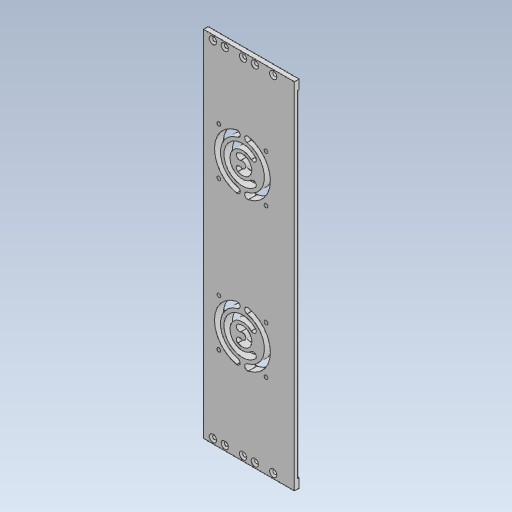
# Autodesk Inventor part: rIGHTbOXcOVER
Saved by Autodesk Inventor 2020 (Build 240168000, 168)
## iProperties
Created: 2019-06-04
Part Number: rIGHTbOXcOVER
Material: Generic
Document SubType Name: Modeling
Designer: LillaHunden
Density: 1 g/cm^3
Appearance: Default
Author: LillaHunden
Autodesk Inventor part; units mm, degrees
ref_plane "YZ Plane" through (0, 0, 0) normal (1, 0, 0) x (0, 1, 0)
ref_plane "XZ Plane" through (0, 0, 0) normal (0, 1, 0) x (-1, 0, 0)
sketch "Sketch1" plane through (0, 0, 0) normal (0, 0, 1) x (1, 0, 0)
  line L0 (0, -288) -> (0, 12) projected
  line L1 (0, 12) -> (76.9823, 12) projected
  line L2 (76.9823, 12) -> (76.9823, -288) projected
  line L3 (76.9823, -288) -> (0, -288) projected
  circle A0 centre (18, -283.95) radius 3.15 projected
  circle A1 centre (43.4912, -283.95) radius 3.15 projected
  circle A2 centre (68.9823, -283.95) radius 3.15 projected
  circle A3 centre (58.9823, -283.95) radius 3.15 projected
  circle A4 centre (33.4912, -283.95) radius 3.15 projected
  circle A5 centre (8, -283.95) radius 3.15 projected
  circle A6 centre (18, 7.95) radius 3.15 projected
  circle A7 centre (43.4912, 7.95) radius 3.15 projected
  circle A8 centre (68.9823, 7.95) radius 3.15 projected
  circle A9 centre (33.4912, 7.95) radius 3.15 projected
  circle A10 centre (8, 7.95) radius 3.15 projected
  circle A11 centre (58.9823, 7.95) radius 3.15 projected
  circle A12 centre (51.5, -236.7541) radius 3.15 projected
  circle A13 centre (51.5, -186.7541) radius 3.15 projected
  circle A14 centre (61.5, -161.7541) radius 3.15 projected
  circle A15 centre (61.5, -186.7541) radius 3.15 projected
  circle A16 centre (61.5, -211.7541) radius 3.15 projected
  circle A17 centre (51.5, -161.7541) radius 3.15 projected
  circle A18 centre (51.5, -211.7541) radius 3.15 projected
  circle A19 centre (51.5, -261.7541) radius 3.15 projected
  point P0 (0, 0)
extrude "Extrusion1" add sketch "Sketch1" along normal blind 12 contours L0 L1 L2 L3 | A0 | A1 | A2 | A3 | A4 | A5 | A6 | A7 | A8 | A9 | A10 | A11 | A12 | A13 | A14 | A15 | A16 | A17 | A18 | A19
sketch "Sketch2" plane through (0, 0, 0) normal (0, 0, -1) x (-1, 0, 0)
  line L0 (-67, 4) -> (-76.9823, 4) construction
  line L1 (-76.9823, -280) -> (-76.9823, 4) construction
  line L2 (-67, -280) -> (-76.9823, -280) construction
  line L3 (-67, 4) -> (-67, -280) construction
  line L4 (-66.8, -280.2) -> (-77.1823, -280.2)
  line L5 (-77.1823, -280.2) -> (-77.1823, 4.2)
  line L6 (-77.1823, 4.2) -> (-66.8, 4.2)
  line L7 (-66.8, 4.2) -> (-66.8, -280.2)
  point P0 (0, 0)
  dimension "d2" = 0.2
  constraints: 8 end point, 3 other
  measures "d2" distance between parallel lines of L3 L7
extrude "Extrusion2" cut sketch "Sketch2" against normal blind 9.25
sketch "Sketch3" plane through (0, 0, 0) normal (0, 0, -1) x (-1, 0, 0)
  line L0 (0, -276) -> (-67, -276) construction
  line L1 (-76.9823, -288) -> (0, -288) construction
  line L2 (-76.9823, -280) -> (-76.9823, -288) construction
  line L3 (-67, -280) -> (-67, 4) construction
  line L4 (-76.9823, -288) -> (0, -288)
  line L5 (0, -288) -> (0, -275.8)
  line L6 (0, -275.8) -> (-76.9823, -275.8)
  line L7 (-76.9823, -275.8) -> (-76.9823, -288)
  line L8 (0, 12) -> (0, -288) projected
  point P0 (0, 0)
  point P1 (0, -281.9)
  dimension "d5" = 0.2
  constraints: 8 end point, 2 parallel, 1 horizontal, 1 midpoint, 1 perpendicular, 1 point on line
  measures "d5" distance between parallel lines of L0 L6
extrude "Extrusion3" cut sketch "Sketch3" against normal blind 8.05
sketch "Sketch4" plane through (66.8, -280.2, 9.25) normal (1, 0, 0) x (0, 0, -1)
  line L0 (1.2, 4.4) -> (9.25, 4.4) construction
  line L1 (9.25, 284.4) -> (9.25, 4.4) construction
  line L2 (9.25, 284.4) -> (0, 284.4) projected
  line L3 (0, 284.4) -> (0, 0) projected
  line L4 (1.2, 0) -> (0, 0) projected
  line L5 (1.2, 0) -> (1.2, 4.4) projected
  line L6 (1.25, 284.2) -> (1.25, 0.2) projected
  line L7 (1.25, 284.2) -> (1.25, 284.4)
  line L8 (0, 284.4) -> (1.2, 284.4)
  line L9 (1.2, 284.4) -> (1.2, 0)
  line L10 (1.2, 0) -> (0, 0)
  line L11 (0, 0) -> (0, 284.4)
  point P0 (9.25, 280.2)
  constraints: 10 end point, 2 parallel, 2 perpendicular, 1 horizontal, 1 point on line
extrude "Extrusion4" add sketch "Sketch4" along normal blind 9
sketch "Sketch5" plane through (0, 0, 0) normal (0, 0, -1) x (-1, 0, 0)
  line L0 (0, 0) -> (-67, 0) construction
  line L1 (-75.8, 4.2) -> (-66.8, 4.2) construction
  line L2 (-66.8, 4.2) -> (-66.8, -275.8) construction
  line L3 (-76.9823, 4.2) -> (-66.8, 4.2) construction
  line L4 (-76.9823, 4.2) -> (-76.9823, 12) construction
  line L5 (-76.9823, 12) -> (0, 12) construction
  line L6 (0, 12) -> (0, -275.8) construction
  line L7 (0, -0.2) -> (-67, -0.2)
  line L8 (-76.9823, 12) -> (0, 12)
  line L9 (0, 12) -> (0, -0.2)
  line L10 (0, -0.2) -> (-76.9823, -0.2)
  line L11 (-76.9823, -0.2) -> (-76.9823, 12)
  dimension "d10" = 0.2
  constraints: 10 end point, 3 parallel, 1 horizontal, 1 perpendicular
  measures "d10" distance between parallel lines of L0 L7
ref_plane "Work Plane1" through (0, 0, 8) normal (0, 0, 1) x (1, 0, 0)
extrude "Extrusion5" cut sketch "Sketch5" against normal up to surface (8 mm away)
sketch "Sketch6" plane through (0, -0.2, 0) normal (0, 1, 0) x (1, 0, 0)
  point P0 (56.9823, -3)
  point P1 (46.9823, -3)
  point P2 (30, -3)
  point P3 (20, -3)
hole "Hole1" at (56.9823, -0.2, 3) at (46.9823, -0.2, 3) at (30, -0.2, 3) at (20, -0.2, 3) direction (0, -1, 0) diameter 2.459 depth 8 tip angle 120 thread size "M3x0.5" class "6H" standard "ISO Metric profile"
sketch "Sketch7" plane through (0, 0, 12) normal (0, 0, 1) x (1, 0, 0)
  circle A0 centre (68.9823, 7.95) radius 3.15 construction
  circle A1 centre (58.9823, 7.95) radius 3.15 construction
  circle A2 centre (43.4912, 7.95) radius 3.15 construction
  circle A3 centre (33.4912, 7.95) radius 3.15 construction
  circle A4 centre (18, 7.95) radius 3.15 construction
  circle A5 centre (8, 7.95) radius 3.15 construction
  circle A6 centre (8, -283.95) radius 3.15 construction
  circle A7 centre (18, -283.95) radius 3.15 construction
  circle A8 centre (33.4912, -283.95) radius 3.15 construction
  circle A9 centre (43.4912, -283.95) radius 3.15 construction
  circle A10 centre (58.9823, -283.95) radius 3.15 construction
  circle A11 centre (68.9823, -283.95) radius 3.15 construction
  point P0 (0, 0)
sketch "Sketch9" plane through (0, 0, 12) normal (0, 0, 1) x (1, 0, 0)
  point P0 (8, 7.95)
  point P1 (18, 7.95)
  point P2 (33.4912, 7.95)
  point P3 (43.4912, 7.95)
  point P4 (58.9823, 7.95)
hole "Hole4" at (8, 7.95, 12) at (18, 7.95, 12) at (33.4912, 7.95, 12) at (43.4912, 7.95, 12) at (58.9823, 7.95, 12) direction (0, 0, -1) diameter 3.4 depth 4 countersink diameter 6.3 countersink angle 90
sketch "Sketch10" plane through (0, 0, 12) normal (0, 0, 1) x (1, 0, 0)
  point P0 (58.9823, -283.95)
  point P1 (43.4912, -283.95)
  point P2 (33.4912, -283.95)
  point P3 (18, -283.95)
  point P4 (8, -283.95)
hole "Hole6" at (58.9823, -283.95, 12) at (43.4912, -283.95, 12) at (33.4912, -283.95, 12) at (18, -283.95, 12) at (8, -283.95, 12) direction (0, 0, -1) diameter 3.4 depth 3.95 countersink diameter 6.3 countersink angle 90
sketch "Sketch11" plane through (0, 0, 12) normal (0, 0, 1) x (1, 0, 0)
  line L0 (53, -176.5677) -> (13, -176.5677) construction
  line L1 (13, -176.5677) -> (13, -216.5677) construction
  line L2 (13, -216.5677) -> (53, -216.5677) construction
  line L3 (53, -216.5677) -> (53, -176.5677) construction
  line L4 (53, -50.8348) -> (13, -50.8348) construction
  line L5 (13, -50.8348) -> (13, -90.8348) construction
  line L6 (13, -90.8348) -> (53, -90.8348) construction
  line L7 (53, -90.8348) -> (53, -50.8348) construction
  line L8 (0, 12) -> (0, -288) projected
  point P0 (0, 0)
  point P1 (53, -70.8348)
  point P2 (53, -196.5677)
  dimension "d41" = 40
  dimension "d42" = 40
  dimension "d43" = 40
  dimension "d44" = 40
  dimension "d45" = 13
  constraints: 16 end point, 8 coincident, 4 parallel, 2 horizontal, 2 midpoint, 2 perpendicular, 1 vertical alignment
  measures "d41" distance of L2.end L1.end
  measures "d42" distance of L1.end L0.end
  measures "d43" distance of L6.end L5.end
  measures "d44" distance of L5.end L4.end
  measures "d45" distance between parallel lines of L8 L5
hole "Hole8" at (13, -176.5677, 12) at (13, -216.5677, 12) at (53, -216.5677, 12) at (53, -176.5677, 12) at (13, -50.8348, 12) at (13, -90.8348, 12) at (53, -90.8348, 12) at (53, -50.8348, 12) direction (0, 0, -1) diameter 3.242 end through all thread size "M4x0.7" class "6H" standard "ISO Metric profile"
sketch "Sketch12" plane through (0, 0, 12) normal (0, 0, 1) x (1, 0, 0)
  circle A0 centre (53, -90.8348) radius 1.621 construction
  circle A1 centre (13, -50.8348) radius 1.621 construction
  circle A2 centre (53, -216.5677) radius 1.621 construction
  circle A3 centre (13, -176.5677) radius 1.621 construction
  circle A4 centre (13, -216.5677) radius 1.621 construction
  circle A5 centre (53, -176.5677) radius 1.621 construction
  circle A6 centre (13, -90.8348) radius 1.621 construction
  circle A7 centre (53, -50.8348) radius 1.621 construction
  circle A8 centre (18, -283.95) radius 3.15 construction
  circle A9 centre (43.4912, -283.95) radius 3.15 construction
  circle A10 centre (58.9823, -283.95) radius 3.15 construction
  circle A11 centre (33.4912, -283.95) radius 3.15 construction
  circle A12 centre (8, -283.95) radius 3.15 construction
  circle A13 centre (43.4912, 7.95) radius 3.15 construction
  circle A14 centre (18, 7.95) radius 3.15 construction
  circle A15 centre (8, 7.95) radius 3.15 construction
  circle A16 centre (33.4912, 7.95) radius 3.15 construction
  circle A17 centre (58.9823, 7.95) radius 3.15 construction
  line L0 (76.9823, 12) -> (0, 12) construction
  line L1 (0, 12) -> (0, -288) construction
  line L2 (0, -288) -> (76.9823, -288) construction
  line L3 (76.9823, -288) -> (76.9823, 12) construction
  line L4 (53, -90.8348) -> (13, -50.8348) construction
  line L5 (13, -50.8348) -> (53, -50.8348) construction
  line L6 (53, -50.8348) -> (13, -90.8348) construction
  line L7 (13, -176.5677) -> (13, -216.5677) construction
  line L8 (13, -216.5677) -> (53, -216.5677) construction
  line L9 (53, -216.5677) -> (13, -176.5677) construction
  line L10 (53, -176.5677) -> (13, -216.5677) construction
  circle A18 centre (33, -70.8348) radius 24 construction
  circle A19 centre (33, -196.5677) radius 24 construction
  arc A20 (37.3584, -91.5413) -> (37.3584, -50.1283) centre (33, -70.8348) ccw construction
  arc A21 (37.8806, -94.0225) -> (37.8806, -47.647) centre (33, -70.8348) ccw
  arc A22 (36.8361, -89.06) -> (36.8361, -52.6095) centre (33, -70.8348) ccw
  arc A23 (36.8361, -89.06) -> (37.8806, -94.0225) centre (37.3584, -91.5413) ccw
  arc A24 (37.8806, -47.647) -> (36.8361, -52.6095) centre (37.3584, -50.1283) ccw
  arc A25 (42.3123, -61.5224) -> (42.3123, -80.1471) centre (33, -70.8348) ccw construction
  arc A26 (44.1052, -59.7295) -> (44.1052, -81.94) centre (33, -70.8348) ccw
  arc A27 (40.5194, -63.3154) -> (40.5194, -78.3541) centre (33, -70.8348) ccw
  arc A28 (40.5194, -63.3154) -> (44.1052, -59.7295) centre (42.3123, -61.5224) ccw
  arc A29 (44.1052, -81.94) -> (40.5194, -78.3541) centre (42.3123, -80.1471) ccw
  line L11 (33, -43.5046) -> (33, -109.6187) construction
  line L12 (53, -50.8348) -> (13, -50.8348) construction
  circle A30 centre (33, -70.8348) radius 24 construction
  arc A31 (28.6416, -50.1283) -> (28.6416, -91.5413) centre (33, -70.8348) ccw construction
  arc A32 (28.1194, -47.647) -> (28.1194, -94.0225) centre (33, -70.8348) ccw
  arc A33 (29.1639, -52.6095) -> (29.1639, -89.06) centre (33, -70.8348) ccw
  arc A34 (28.1194, -94.0225) -> (29.1639, -89.06) centre (28.6416, -91.5413) ccw
  arc A35 (29.1639, -52.6095) -> (28.1194, -47.647) centre (28.6416, -50.1283) ccw
  arc A36 (30.3412, -75.5506) -> (30.3412, -66.1189) centre (33, -70.8348) ccw construction
  arc A37 (29.0751, -77.7962) -> (29.0751, -63.8734) centre (33, -70.8348) ccw
  arc A38 (31.6072, -73.3051) -> (31.6072, -68.3644) centre (33, -70.8348) ccw
  arc A39 (31.6072, -73.3051) -> (29.0751, -77.7962) centre (30.3412, -75.5506) ccw
  arc A40 (29.0751, -63.8734) -> (31.6072, -68.3644) centre (30.3412, -66.1189) ccw
  arc A41 (28.1194, -219.7555) -> (29.1639, -214.793) centre (28.6416, -217.2743) ccw
  arc A42 (44.1052, -207.673) -> (40.5194, -204.0871) centre (42.3123, -205.8801) ccw
  arc A43 (29.0751, -203.5292) -> (29.0751, -189.6064) centre (33, -196.5678) ccw
  arc A44 (29.0751, -189.6064) -> (31.6072, -194.0974) centre (30.3412, -191.8519) ccw
  arc A45 (40.5194, -189.0484) -> (40.5194, -204.0871) centre (33, -196.5678) ccw
  arc A46 (37.8806, -173.38) -> (36.8361, -178.3425) centre (37.3584, -175.8613) ccw
  arc A47 (42.3123, -187.2554) -> (42.3123, -205.8801) centre (33, -196.5678) ccw construction
  arc A48 (29.1639, -178.3425) -> (28.1194, -173.38) centre (28.6416, -175.8613) ccw
  arc A49 (36.8361, -214.793) -> (36.8361, -178.3425) centre (33, -196.5678) ccw
  arc A50 (44.1052, -185.4625) -> (44.1052, -207.673) centre (33, -196.5678) ccw
  arc A51 (37.3584, -217.2743) -> (37.3584, -175.8613) centre (33, -196.5678) ccw construction
  arc A52 (29.1639, -178.3425) -> (29.1639, -214.793) centre (33, -196.5678) ccw
  arc A53 (37.8806, -219.7555) -> (37.8806, -173.38) centre (33, -196.5678) ccw
  line L13 (13, -176.5678) -> (53, -176.5678) construction
  line L14 (53, -176.5678) -> (13, -176.5678) construction
  line L15 (53, -216.5678) -> (13, -176.5678) construction
  line L16 (53, -176.5678) -> (13, -216.5678) construction
  circle A54 centre (33, -196.5678) radius 24 construction
  circle A55 centre (33, -196.5678) radius 24 construction
  arc A56 (28.6416, -175.8613) -> (28.6416, -217.2743) centre (33, -196.5678) ccw construction
  arc A57 (28.1194, -173.38) -> (28.1194, -219.7555) centre (33, -196.5678) ccw
  arc A58 (40.5194, -189.0484) -> (44.1052, -185.4625) centre (42.3123, -187.2554) ccw
  arc A59 (31.6072, -199.0381) -> (31.6072, -194.0974) centre (33, -196.5678) ccw
  arc A60 (30.3412, -201.2836) -> (30.3412, -191.8519) centre (33, -196.5678) ccw construction
  arc A61 (31.6072, -199.0381) -> (29.0751, -203.5292) centre (30.3412, -201.2836) ccw
  arc A62 (36.8361, -214.793) -> (37.8806, -219.7555) centre (37.3584, -217.2743) ccw
  point P0 (0, 0)
  point P1 (33, -169.2376)
  dimension "d53" = 48
  dimension "d54" = 48
  dimension "d55" = 2.5356
  dimension "d56" = 2.5356
  dimension "d59" = 125.733
  dimension "d62" = 125.733
  constraints: 80 point on circle, 45 centre point, 26 end point, 12 tangent, 8 coincident, 8 symmetric about line, 4 vertical alignment, 3 perpendicular, 3 vertical, 2 midpoint, 2 point on line, 1 horizontal, 67 other
  measures "d53" diameter of A18
  measures "d54" diameter of A19
  measures "d55" radius of A29
  measures "d56" radius of A23
  measures "d59" distance of A18.centre A19.centre
  measures "d62" distance of A34.centre A41.centre
extrude "Extrusion6" cut sketch "Sketch12" against normal through all
sketch "Sketch13" plane through (0, 0, 0) normal (0, 0, -1) x (-1, 0, 0)
  line L0 (-58, -98.3348) -> (-8, -98.3348)
  line L1 (-5.5, -95.8348) -> (-5.5, -45.8348)
  line L2 (-8, -43.3348) -> (-58, -43.3348)
  line L3 (-60.5, -45.8348) -> (-60.5, -95.8348)
  arc A0 (-31.6072, -68.3644) -> (-31.6072, -73.3051) centre (-33, -70.8348) ccw construction
  arc A1 (-60.5, -95.8348) -> (-58, -98.3348) centre (-58, -95.8348) ccw
  arc A2 (-58, -43.3348) -> (-60.5, -45.8348) centre (-58, -45.8348) ccw
  arc A3 (-5.5, -45.8348) -> (-8, -43.3348) centre (-8, -45.8348) ccw
  arc A4 (-8, -98.3348) -> (-5.5, -95.8348) centre (-8, -95.8348) ccw
  line L4 (-33, -70.8348) -> (-50.7028, -70.8348) construction
  arc A5 (-8, -224.0678) -> (-5.5, -221.5678) centre (-8, -221.5678) ccw
  line L5 (-58, -224.0678) -> (-8, -224.0678)
  arc A6 (-60.5, -221.5678) -> (-58, -224.0678) centre (-58, -221.5678) ccw
  line L6 (-5.5, -221.5678) -> (-5.5, -171.5678)
  line L7 (-33, -196.5678) -> (-50.7028, -196.5678) construction
  arc A7 (-5.5, -171.5678) -> (-8, -169.0678) centre (-8, -171.5678) ccw
  line L8 (-8, -169.0678) -> (-58, -169.0678)
  line L9 (-60.5, -171.5678) -> (-60.5, -221.5678)
  arc A8 (-58, -169.0678) -> (-60.5, -171.5678) centre (-58, -171.5678) ccw
  point P0 (0, 0)
  point P1 (-5.5, -43.3348)
  point P2 (-5.5, -98.3348)
  point P3 (-60.5, -43.3348)
  point P4 (-60.5, -70.8348)
  point P5 (-33, -43.3348)
  point P6 (-5.5, -224.0678)
  point P7 (-31.6072, -199.0381)
  point P8 (-31.6072, -194.0974)
  point P9 (-5.5, -169.0678)
  point P10 (-33, -169.0678)
  point P11 (-60.5, -169.0678)
  point P12 (-60.5, -196.5678)
  dimension "d67" = 55
  dimension "d68" = 55
  dimension "d69" = 2.5
  dimension "d72" = 125.733
  constraints: 20 end point, 16 point on circle, 12 point on line, 8 centre point, 8 tangent, 3 equal radius, 2 horizontal, 2 midpoint, 2 parallel, 1 collinear, 1 horizontal alignment, 1 perpendicular, 1 vertical, 1 vertical alignment, 29 other
  measures "d67" distance of point (-5.5, -43.335) point (-60.5, -43.335)
  measures "d68" distance of point (-5.5, -98.335) point (-5.5, -43.335)
  measures "d69" radius of A1
  measures "d72" distance of L1.start L6.start
extrude "Extrusion7" cut sketch "Sketch13" against normal blind 4.75
move faces "Move1" translate (0, 0, -0.05) faces at (72.8, -183.9333, 8.05)
equation "\"d56\" = d55"
equation "\"d68\" = d67"
body "Solid1"
